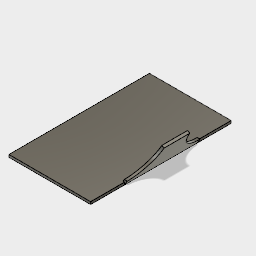
LIDAR Enclosure Lid v2 (Autodesk Fusion 360 design; units mm, degrees)
Autodesk Fusion 360 part; units mm, degrees
note: some values were not read from the file. Set by a fixed rule: which sketch regions a step uses.
sketch "Sketch2" plane through (0, 0, 0) normal (0, 1, 0) x (1, 0, 0)
  line L0 (0, 0) -> (55, 0)
  line L1 (55, 0) -> (55, 32)
  line L2 (55, 32) -> (0, 32)
  line L3 (0, 32) -> (0, 0)
  dimension "d5" = 55
  dimension "d6" = 32
  constraint horizontal L0
  constraint vertical L1
  constraint horizontal L2
  constraint vertical L3
  constraint coincident L0.start L3.end
extrude "Extrude2" add sketch "Sketch2" along normal blind 1
ref_plane "WorkPlane1" through (12.125, 0, 0) normal (0, 0.492424, -0.870356) x (1, 0, 0)
sketch "Sketch3" plane through (12.125, 0, 0) normal (0, 0.492424, -0.870356) x (1, 0, 0)
  line L0 (1.151, -0.8704) -> (1.151, -3.4842)
  line L1 (10.0729, -12.68) -> (20.4753, -12.68)
  line L2 (29.599, -3.4803) -> (29.599, -0.8704)
  line L3 (-12.125, -0.8704) -> (42.875, -0.8704)
  line L4 (42.875, -0.8704) -> (42.875, 14.8872)
  line L5 (-12.125, 14.8872) -> (-12.125, -0.8704)
  line L6 (-12.125, 0) -> (38, 0)
  line L7 (1.151, -0.8704) -> (1.151, 0)
  line L8 (29.599, -0.8704) -> (29.599, 0)
  line L9 (29.599, -0.8704) -> (10.0729, -0.8704)
  line L10 (10.0729, -12.68) -> (29.599, -12.68)
  line L11 (29.599, -12.68) -> (29.599, -0.8704)
  line L12 (10.0729, -12.68) -> (1.151, -12.68)
  line L13 (1.151, -12.68) -> (1.151, -0.8704)
  line L14 (1.151, -0.8704) -> (10.0729, -0.8704)
  dimension "d10" = 13.276
  dimension "d11" = 13.276
  dimension "d17" = 12.68
  constraint vertical L0
  constraint horizontal L1
  constraint vertical L2
  constraint coincident origin L3
  constraint coincident L5 origin
  constraint perpendicular L5 L6
  constraint coincident L6 origin
  constraint perpendicular L6 L7
  constraint perpendicular L6 L8
  constraint horizontal L9
  constraint horizontal L10
  constraint vertical L11
  constraint horizontal L12
  constraint vertical L13
  constraint horizontal L14
  measures "d10" distance of L2 L4
  measures "d11" distance of L0 L5
  measures "d17" distance of L1 L6
extrude "Extrude4" add sketch "Sketch3" along normal blind 1 contours L0 L1 L2 L3 L9 L10 L11 L12 L13 L14 | L3 L6 L7 L8 L9 L14
sketch "Sketch4" plane through (0, 0, -32) normal (0, 0, -1) x (-1, 0, 0)
  line L0 (-55, 0) -> (0, 0)
  line L1 (0, 0) -> (0, 1)
  line L2 (0, 1) -> (-55, 1)
  line L3 (-55, 1) -> (-55, 0)
  circle A0 centre (-41.724, 11.0361) radius 9.2
  circle A1 centre (-13.276, 11.0361) radius 9.2
  dimension "d22" = 18.4
  dimension "d23" = 18.4
  constraint coincident L0.end L1.start
  measures "d22" diameter of A0
  measures "d23" diameter of A1
extrude "Extrude5" cut sketch "Sketch4" against normal blind 72 contours A0 | A1
